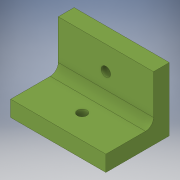
# Autodesk Inventor part: Tension Angle
Saved by Autodesk Inventor 2017 (Build 210142000, 142)
## iProperties
Created: 2017-01-26
Part Number: Tension Angle
Material: Generic
Document SubType Name: Modeling
Designer: Ben
Density: 1 g/cm^3
Appearance: Olive Green
Author: Ben
Autodesk Inventor part; units mm, degrees
ref_plane "YZ Plane" through (0, 0, 0) normal (1, 0, 0) x (0, 1, 0)
ref_plane "XZ Plane" through (0, 0, 0) normal (0, 1, 0) x (-1, 0, 0)
ref_plane "XY Plane" through (0, 0, 0) normal (0, 0, 1) x (1, 0, 0)
sketch "Sketch1" plane through (0, 0, 0) normal (1, 0, 0) x (0, 1, 0)
  line L0 (0, 25.4) -> (0, 0)
  line L1 (0, 0) -> (25.4, 0)
  line L2 (25.4, 0) -> (25.4, 6.35)
  line L3 (25.4, 6.35) -> (9.525, 6.35)
  line L4 (6.35, 9.525) -> (6.35, 25.4)
  line L5 (6.35, 25.4) -> (0, 25.4)
  arc A0 (6.35, 9.525) -> (9.525, 6.35) centre (9.525, 9.525) ccw
  dimension "d0" = 3.175
  dimension "d1" = 25.4
  dimension "d2" = 6.35
  constraints: 12 end point, 7 perpendicular, 2 point on circle, 2 tangent, 1 centre point, 1 vertical
  measures "d0" radius of A0
  measures "d1" distance of L0.end L1.end
  measures "d2" distance of L1.end L2.end
extrude "Extrusion1" add sketch "Sketch1" along normal blind 38.1
sketch "Sketch2" plane through (0, 0, 0) normal (0, 0, -1) x (-1, 0, 0)
  line L0 (0, 6.35) -> (-38.1, 6.35) construction
  line L1 (-19.05, 6.35) -> (-19.05, 25.4) construction
  line L2 (0, 25.4) -> (-38.1, 25.4) construction
  circle A0 centre (-19.05, 15.875) radius 1.905
  point P0 (0, 0)
  dimension "d5" = 3.81
  constraints: 3 midpoint, 2 end point, 1 centre point
  measures "d5" diameter of A0
extrude "Extrusion2" cut sketch "Sketch2" against normal through all
sketch "Sketch3" plane through (0, 0, 0) normal (0, -1, 0) x (1, 0, 0)
  line L0 (0, 6.35) -> (38.1, 6.35) construction
  line L1 (17.145, 6.35) -> (20.955, 6.35) construction
  line L2 (19.05, 6.35) -> (19.05, 25.4) construction
  line L3 (0, 25.4) -> (38.1, 25.4) construction
  circle A0 centre (19.05, 15.875) radius 1.905
  point P0 (0, 0)
  dimension "d8" = 3.81
  constraints: 3 midpoint, 2 end point, 1 centre point
  measures "d8" diameter of A0
extrude "Extrusion3" cut sketch "Sketch3" against normal through all
body "Solid1"
